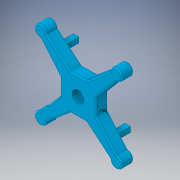
# Autodesk Inventor part: Drone Frame
Saved by Autodesk Inventor 2019 (Build 230136000, 136)
## iProperties
Created: 2019-02-21
Part Number: Drone Frame
Material: Generic
Document SubType Name: Modeling
Designer: k0904676
Density: 1 g/cm^3
Appearance: Sky Blue Medium
Author: k0904676
Autodesk Inventor part; units mm, degrees
ref_plane "YZ Plane" through (0, 0, 0) normal (1, 0, 0) x (0, 1, 0)
ref_plane "XZ Plane" through (0, 0, 0) normal (0, 1, 0) x (-1, 0, 0)
ref_plane "XY Plane" through (0, 0, 0) normal (0, 0, 1) x (1, 0, 0)
sketch "Sketch1" plane through (0, 0, 0) normal (0, 0, 1) x (1, 0, 0)
  line L0 (-34.925, -38.1) -> (34.925, -38.1)
  line L1 (38.1, -34.925) -> (38.1, 34.925)
  line L2 (34.925, 38.1) -> (-34.925, 38.1)
  line L3 (-38.1, 34.925) -> (-38.1, -34.925)
  line L4 (-38.1, -38.1) -> (38.1, 38.1) construction
  line L5 (38.1, -38.1) -> (-38.1, 38.1) construction
  arc A0 (-34.925, 38.1) -> (-38.1, 34.925) centre (-34.925, 34.925) ccw
  arc A1 (-38.1, -34.925) -> (-34.925, -38.1) centre (-34.925, -34.925) ccw
  arc A2 (34.925, -38.1) -> (38.1, -34.925) centre (34.925, -34.925) ccw
  arc A3 (38.1, 34.925) -> (34.925, 38.1) centre (34.925, 34.925) ccw
  circle A4 centre (0, 0) radius 12.7
  line L6 (0, -38.1) -> (17.4625, -38.1)
  line L7 (17.4625, -38.1) -> (80.6655, -80.6655)
  line L8 (38.1, 0) -> (38.1, -17.4625)
  line L9 (38.1, -17.4625) -> (80.6655, -80.6655)
  circle A5 centre (80.6655, -80.6655) radius 12.7
  line L10 (17.4625, -38.1) -> (67.9655, -80.6655)
  line L11 (38.1, -17.4625) -> (80.6655, -67.9655)
  circle A6 centre (80.6655, 80.6655) radius 12.7
  line L12 (38.1, 17.4625) -> (80.6655, 67.9655)
  line L13 (17.4625, 38.1) -> (67.9655, 80.6655)
  circle A7 centre (-80.6655, 80.6655) radius 12.7
  line L14 (-17.4625, 38.1) -> (-67.9655, 80.6655)
  line L15 (-38.1, 17.4625) -> (-80.6655, 67.9655)
  circle A8 centre (-80.6655, -80.6655) radius 12.7
  line L16 (-38.1, -17.4625) -> (-80.6655, -67.9655)
  line L17 (-17.4625, -38.1) -> (-67.9655, -80.6655)
  line L18 (17.4625, -38.1) -> (38.1, -17.4625)
  line L19 (17.4625, 38.1) -> (38.1, 17.4625)
  line L20 (-38.1, -17.4625) -> (-17.4625, -38.1)
  line L21 (-38.1, 17.4625) -> (-17.4625, 38.1)
  dimension "d0" = 76.2
  dimension "d1" = 76.2
  dimension "d2" = 3.175
  dimension "d3" = 25.4
  dimension "d4" = 17.4625
  dimension "d5" = 76.2
  dimension "d6" = 17.4625
  dimension "d7" = 25.4
  dimension "d10" = 360
  constraints: 44 end point, 16 point on circle, 12 point on line, 9 centre point, 8 tangent, 4 midpoint, 3 equal radius, 2 coincident, 2 parallel, 1 horizontal, 1 perpendicular, 33 other
  measures "d0" distance of L5.end L4.end
  measures "d1" distance of L4.end L5.start
  measures "d2" radius of A0
  measures "d3" diameter of A4
  measures "d4" distance of L6.start L6.end
  measures "d5" distance of L6.end L7.end
  measures "d6" distance of L8.start L8.end
  measures "d7" diameter of A5
extrude "Extrusion1" add sketch "Sketch1" along normal blind 25.4
fillet "Fillet1" radius 3.175 31 edges at (42.714, -59.3827, 25.4) (0, -38.1, 25.4) (-42.714, -59.3827, 25.4) (-59.3827, -42.714, 25.4) (-38.1, 0, 25.4) (-59.3827, 42.714, 25.4) (-42.714, 59.3827, 25.4) (-89.6458, 89.6458, 25.4) (-89.6458, -89.6458, 25.4) (89.6458, -89.6458, 25.4) (59.3827, -42.714, 25.4) (38.1, 0, 25.4) (59.3827, 42.714, 25.4) (89.6458, 89.6458, 25.4) (42.714, 59.3827, 25.4) (0, 38.1, 25.4) (38.1, 0, 0) (59.3827, -42.714, 0) (89.6458, -89.6458, 0) (42.714, -59.3827, 0) (0, -38.1, 0) (-42.714, -59.3827, 0) (-89.6458, -89.6458, 0) (-59.3827, -42.714, 0) (-38.1, 0, 0) (-59.3827, 42.714, 0) (-89.6458, 89.6458, 0) (-42.714, 59.3827, 0) (0, 38.1, 0) (42.714, 59.3827, 0) (89.6458, 89.6458, 0)
sketch "Sketch2" plane through (0, 0, 0) normal (0, 0, -1) x (-1, 0, 0)
  point P0 (0, 0)
fillet "Fillet2" radius 3.175 3 edges at (36.5125, 15.579, 0) (59.3827, 42.714, 0) (82.2247, 69.8155, 0)
sketch "Sketch3" plane through (0, 0, 0) normal (0, 0, -1) x (-1, 0, 0)
  line L0 (-34.925, 18.622) -> (-79.2752, 71.2425) projected
  line L1 (-34.925, 18.622) -> (-15.875, 18.622)
  line L2 (-15.875, 18.622) -> (-15.875, -18.622)
  line L3 (-15.875, -18.622) -> (-34.925, -18.622)
  line L4 (-34.925, -18.622) -> (-34.925, 18.622)
  point P0 (0, 0)
  dimension "d16" = 19.05
  constraints: 8 end point, 2 parallel, 1 horizontal, 1 perpendicular
  measures "d16" distance of L2.end L3.end
sketch "Sketch4" plane through (0, 0, 0) normal (0, 1, 0) x (-1, 0, 0)
  point P0 (0, 0)
sketch "Sketch5" plane through (0, 0, 0) normal (0, 0, -1) x (-1, 0, 0)
  line L0 (-79.2752, -71.2425) -> (-34.925, -18.622) projected
  line L1 (-49.1344, -60.8701) -> (-60.8213, -60.8701)
  line L2 (-60.8213, -60.8701) -> (-60.8213, -49.3474)
  line L3 (-60.8213, -49.3474) -> (-49.1344, -49.3474)
  line L4 (-49.1344, -49.3474) -> (-49.1344, -60.8701)
  line L5 (-49.1344, -60.8701) -> (-60.8213, -49.3474) construction
  line L6 (-60.8213, -60.8701) -> (-49.1344, -49.3474) construction
  point P0 (0, 0)
  point P1 (-54.9778, -55.1087)
  constraints: 12 end point, 2 midpoint, 2 parallel, 1 horizontal, 1 perpendicular, 1 point on line
extrude "Extrusion3" add sketch "Sketch5" along normal blind 25.4
pattern_circular "Circular Pattern2" count 4 over 360 about axis through (0, 0, -10) along (0, 0, 1) of "Extrusion3"
body "Solid1"
